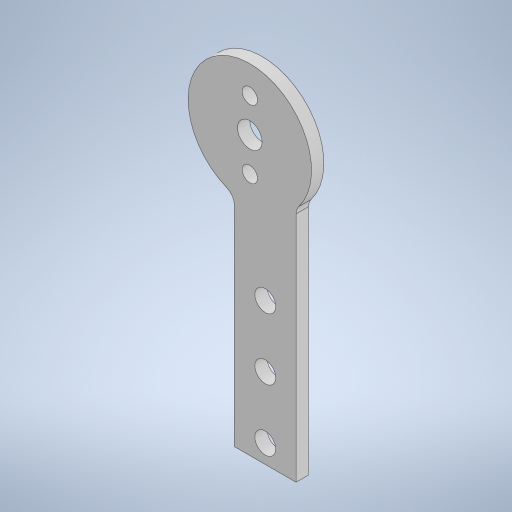
# Autodesk Inventor part: cutter_board_claws_endeffector_8_5_rotary-blade
Saved by Autodesk Inventor 2024 (Build 280153000, 153)
## iProperties
Created: 2025-06-01
Part Number: cutter_board_claws_endeffector_8_5_rotary-blade
Material: 一般
Document SubType Name: Modeling
Designer: 1412z
Density: 1 g/cm^3
Appearance: 既定
Author: 1412z
Autodesk Inventor part; units mm, degrees
ref_plane "YZ Plane" through (0, 0, 0) normal (1, 0, 0) x (0, 1, 0)
ref_plane "XZ Plane" through (0, 0, 0) normal (0, 1, 0) x (-1, 0, 0)
ref_plane "XY Plane" through (0, 0, 0) normal (0, 0, 1) x (1, 0, 0)
sketch "スケッチ1" plane through (0, 0, 0) normal (0, 0, 1) x (1, 0, 0)
  circle A0 centre (0, 0) radius 10
  line L0 (0, 0) -> (7.5, 0)
  line L1 (7.5, 0) -> (7.5, -45)
  line L2 (7.5, -45) -> (-2.5, -45)
  line L3 (-2.5, -45) -> (-2.5, 0)
  circle A1 centre (2.5, -22) radius 1.7
  circle A2 centre (2.5, -32) radius 1.7
  circle A3 centre (2.5, -42) radius 1.7
  circle A4 centre (0, 0) radius 5.5
  circle A5 centre (0, 5.5) radius 1.25
  circle A6 centre (0, -5.5) radius 1.25
  circle A7 centre (0, 0) radius 2
  line L4 (0, 0) -> (0, -45)
  point P0 (7.5, -6.6144)
  point P1 (-2.5, -9.6825)
  dimension "d0" = 20
  dimension "d3" = 7.5
  dimension "d4" = 45
  dimension "d5" = 10
  dimension "d6" = 3.4
  dimension "d7" = 3.4
  dimension "d8" = 3.4
  dimension "d9" = 11
  dimension "d10" = 2.5
  dimension "d11" = 2.5
  dimension "d12" = 4
  dimension "d16" = 2.5
  dimension "d17" = 2.5
  dimension "d18" = 2.5
  constraints: 10 end point, 8 centre point, 4 perpendicular, 3 coincident, 2 point on circle, 2 point on line, 1 horizontal
  measures "d0" diameter of A0
  measures "d3" distance of L0.start L0.end
  measures "d4" distance of L0.end L1.end
  measures "d5" distance of L1.end L2.end
  measures "d6" diameter of A1
  measures "d7" diameter of A2
  measures "d8" diameter of A3
  measures "d9" diameter of A4
  measures "d10" diameter of A5
  measures "d11" diameter of A6
  measures "d12" diameter of A7
  measures "d16" distance from line of L4 A1.centre
  measures "d17" distance from line of L4 A2.centre
  measures "d18" distance from line of L4 A3.centre
extrude "押し出し1" add sketch "スケッチ1" along normal blind 2 contours A0 L1 L0 A4 A5 L3 | L3 A4 A6 L4 A0 | A0 L4 L2 L3 | L1 L2 L4 A0 | A0 L4 A6 A4 L0 L1 | A4 A5 L0 A7 L4 A6 | A4 A6 L4 A7 L0
fillet "フィレット1" radius 2 2 edges at (7.5, -6.6144, 1) (-2.5, -9.6825, 1)
